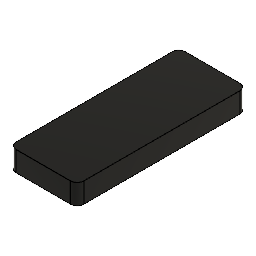
Central Tool Box v19 (Autodesk Fusion 360 archive; units mm, degrees)
design "Soft Spacer"
Autodesk Fusion 360 part; units mm, degrees
sketch "Sketch1" plane through (0, 0, 0) normal (0, 0, 1) x (1, 0, 0)
  line L0 (5, -12.5) -> (-5, -12.5)
  line L1 (-5, -12.5) -> (-5, 12.5)
  line L2 (-5, 12.5) -> (5, 12.5)
  line L3 (5, 12.5) -> (5, -12.5)
  line L4 (5, -12.5) -> (-5, 12.5) construction
  line L5 (-5, -12.5) -> (5, 12.5) construction
  dimension "d1" = 10
  dimension "d2" = 25
  constraint horizontal L0
  constraint perpendicular L0 L1
  constraint parallel L0 L2
  constraint parallel L1 L3
  constraint coincident L4 origin
  constraint coincident L5 origin
  measures "d1" distance of L1.end L2.end
  measures "d2" distance of L0.end L1.end
extrude "Extrude1" add sketch "Sketch1" along normal blind 3
fillet "Fillet1" radius 1 4 edges at (5, -12.5, 1.5) (-5, -12.5, 1.5) (-5, 12.5, 1.5) (5, 12.5, 1.5)

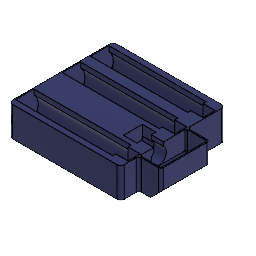
design "CO2 Inflator Holder"
Autodesk Fusion 360 part; units mm, degrees
sketch "Sketch1" plane through (0, 0, 0) normal (0, 0, 1) x (1, 0, 0)
  line L0 (44.5, -42.5) -> (-44.5, -42.5)
  line L1 (-44.5, -42.5) -> (-44.5, 42.5)
  line L2 (-44.5, 42.5) -> (44.5, 42.5)
  line L3 (44.5, 42.5) -> (44.5, -42.5)
  line L4 (44.5, -42.5) -> (-44.5, 42.5) construction
  line L5 (-44.5, -42.5) -> (44.5, 42.5) construction
  dimension "d1" = 85
  dimension "d2" = 89
  constraint horizontal L0
  constraint perpendicular L0 L1
  constraint parallel L0 L2
  constraint parallel L1 L3
  constraint coincident L4 origin
  constraint coincident L5 origin
  measures "d1" distance of L0.end L1.end
  measures "d2" distance of L1.end L2.end
extrude "Extrude1" add sketch "Sketch1" against normal blind 1.2
sketch "Sketch2" plane through (-44.5, 0, 0) normal (-1, 0, 0) x (0, -1, 0)
  line L0 (42.5, 0) -> (-42.5, 0)
  line L1 (-42.5, 0) -> (-42.5, -1.2)
  line L2 (-42.5, -1.2) -> (42.5, -1.2)
  line L3 (42.5, -1.2) -> (42.5, 0)
  line L4 (42.5, 0) -> (42.5, 23.3)
  circle A0 centre (30.5, 11) radius 11
  circle A1 centre (-7.5, 11) radius 11
  circle A2 centre (-30.5, 11) radius 11
  line L5 (38, 23.3) -> (38, 19.0467)
  line L6 (23, 19.0467) -> (23, 23.3)
  line L7 (0, 23.3) -> (0, 19.0467)
  line L8 (-15, 19.0467) -> (-15, 23.3)
  line L9 (-23, 23.3) -> (-23, 19.0467)
  line L10 (-42.5, 0) -> (-42.5, 23.3)
  line L11 (-38, 23.3) -> (-38, 19.0467)
  line L12 (-42.5, 23.3) -> (42.5, 23.3)
  dimension "d5" = 22
  dimension "d7" = 12
  dimension "d10" = 12
  dimension "d12" = 15
  dimension "d17" = 24.5
  dimension "d53" = 38
  constraint coincident L0.start L3.end
  constraint perpendicular L0 L4
  constraint tangent L0 A0
  constraint coincident A0 L5.end
  constraint coincident A0 L6.start
  constraint coincident A1 L7.end
  constraint equal A0 A1
  constraint equal A0 A2
  constraint tangent L0 A1
  constraint tangent L0 A2
  constraint coincident A1 L8.start
  constraint coincident A2 L9.end
  constraint coincident L0.end L1.start
  constraint perpendicular L0 L10
  constraint coincident A2 L11.end
  constraint equal L9 L11
  constraint equal L8 L11
  constraint equal L7 L8
  constraint equal L6 L7
  constraint equal L5 L6
  constraint perpendicular L4 L12
  constraint coincident L5.start L12
  constraint coincident L6.end L12
  constraint coincident L7.start L12
  constraint coincident L8.end L12
  constraint coincident L9.start L12
  constraint coincident L11.start L12
  constraint vertical L5
  constraint vertical L7
  constraint vertical L8
  constraint vertical L9
  constraint vertical L11
  measures "d5" diameter of A0
  measures "d7" distance of L4 A0.centre
  measures "d10" distance of A2.centre L10
  measures "d12" distance of L5 L6
  measures "d17" distance of L2 L12
  measures "d53" distance of A0.centre A1.centre
extrude "Extrude3" add sketch "Sketch2" along normal blind 1
extrude "Extrude4" add sketch "Sketch2" against normal blind 79 contours L0 L4 A0 L5 L12 | L0 A0 A1 L6 L7 L12 | L0 A1 A2 L8 L9 L12 | L0 A2 L10 L11 L12
sketch "Sketch4" plane through (44.5, 0, 0) normal (1, 0, 0) x (0, 1, 0)
  line L0 (42.5, 0) -> (-42.5, 0)
  line L1 (-42.5, 0) -> (-42.5, -1.2)
  line L2 (-42.5, -1.2) -> (42.5, -1.2)
  line L3 (42.5, -1.2) -> (42.5, 0)
  arc A0 (23, 19.0467) -> (30.5, 0) centre (30.5, 11) ccw construction
  arc A1 (30.5, 0) -> (38, 19.0467) centre (30.5, 11) ccw construction
  arc A2 (0, 19.0467) -> (7.5, 0) centre (7.5, 11) ccw construction
  arc A3 (7.5, 0) -> (15, 19.0467) centre (7.5, 11) ccw construction
  arc A4 (-38, 19.0467) -> (-30.5, 0) centre (-30.5, 11) ccw construction
  arc A5 (-30.5, 0) -> (-23, 19.0467) centre (-30.5, 11) ccw construction
  circle A6 centre (30.5, 11) radius 5
  circle A7 centre (7.5, 11) radius 5
  circle A8 centre (-30.5, 11) radius 5
  line L4 (42.5, 0) -> (42.5, 23.3)
  line L5 (-42.5, 23.3) -> (-42.5, 0)
  line L6 (-38, 23.3) -> (-23, 23.3)
  line L7 (-42.5, 23.3) -> (-38, 23.3)
  line L8 (42.5, 23.3) -> (-42.5, 23.3)
  line L9 (-23, 23.3) -> (0, 23.3)
  line L10 (15, 23.3) -> (23, 23.3)
  line L11 (38, 23.3) -> (42.5, 23.3)
  line L12 (35.5, 11) -> (35.5, 27)
  line L13 (25.5, 11) -> (25.5, 27)
  line L14 (12.5, 11) -> (12.5, 23.3)
  line L15 (2.5, 11) -> (2.5, 27)
  line L16 (-25.5, 11) -> (-25.5, 23.3)
  line L17 (-35.5, 11) -> (-35.5, 23.3)
  circle A9 centre (-11.5, 15.05) radius 7.75
  line L18 (-19.25, 15.05) -> (-19.25, 23.3)
  line L19 (-3.75, 15.05) -> (-3.75, 27)
  arc A10 (23, 19.0467) -> (38, 19.0467) centre (30.5, 11) ccw
  arc A11 (0, 19.0467) -> (15, 19.0467) centre (7.5, 11) ccw
  arc A12 (-38, 19.0467) -> (-23, 19.0467) centre (-30.5, 11) ccw
  line L20 (0, 23.3) -> (15, 23.3)
  line L21 (23, 23.3) -> (38, 23.3)
  line L22 (-30.5, 11) -> (7.5, 11) construction
  line L23 (-11.5, 11) -> (-11.5, 15.05) construction
  point P0 (38, 19.0467)
  point P1 (-38, 19.0467)
  point P2 (-23, 19.0467)
  point P3 (38, 19.0467)
  point P4 (-38, 19.0467)
  point P5 (38, 19.0467)
  point P6 (-38, 19.0467)
  dimension "d23" = 10
  dimension "d28" = 15.5
  dimension "d29" = 8.25
  constraint equal A7 A8
  constraint equal A6 A7
  constraint coincident L0.start L3.end
  constraint perpendicular L0 L4
  constraint coincident L0.end L1.start
  constraint coincident L4.end L8.start
  constraint coincident L5.start L7.start
  constraint coincident A6 L12.start
  constraint coincident A6 L13.start
  constraint coincident A7 L14.start
  constraint coincident L6 L14.end
  constraint coincident A7 L15.start
  constraint coincident A8 L16.start
  constraint coincident L6 L16.end
  constraint coincident A8 L17.start
  constraint coincident L6 L17.end
  constraint tangent A6 L13
  constraint tangent A6 L12
  constraint tangent A7 L14
  constraint tangent A7 L15
  constraint tangent A8 L16
  constraint tangent A8 L17
  constraint vertical L17
  constraint vertical L16
  constraint vertical L15
  constraint vertical L14
  constraint vertical L13
  constraint vertical L12
  constraint coincident A9 L18.start
  constraint coincident L6 L18.end
  constraint coincident A9 L19.start
  constraint tangent A9 L19
  constraint tangent A9 L18
  constraint perpendicular L10 L18
  constraint perpendicular L10 L19
  constraint coincident A0.centre A1.centre
  constraint coincident A4.centre A5.centre
  constraint coincident A2.centre A3.centre
  constraint midpoint L22 L23.start
  constraint coincident A9.centre L23.end
  constraint perpendicular L22 L23
  measures "d23" diameter of A6
  measures "d28" diameter of A9
  measures "d29" distance of L6 A9.centre
extrude "Extrude5" add sketch "Sketch4" along normal blind 1
extrude "Extrude6" add sketch "Sketch4" against normal up to surface (10 mm away) contours L0 A6 A7 A8 L4 L5 L6 L7 L8 L9 L10 L11 L12 L13 L14 L15 L16 L17 A9 L18 L19 L20 L21 | L8 L9 A9 L18 L19
extrude "Extrude7" cut sketch "Sketch4" against normal blind 20 contours L8 L9 A9 L18 L19 | A9
sketch "Sketch5" plane through (0, 0, 23.3) normal (0, 0, 1) x (-1, 0, 0)
  line L0 (-44.5, 25.5) -> (-44.5, 35.5)
  line L1 (-45.5, -42.5) -> (45.5, -42.5)
  line L2 (44.5, 38) -> (44.5, 23)
  line L3 (45.5, 42.5) -> (-45.5, 42.5)
  line L4 (-24.5, 19.25) -> (-24.5, 3.75)
  line L5 (-45.5, 42.5) -> (-45.5, -42.5)
  line L6 (-44.5, 35.5) -> (-34.5, 35.5)
  line L7 (-34.5, 35.5) -> (-34.5, 38)
  line L8 (-34.5, 38) -> (44.5, 38)
  line L9 (45.5, -42.5) -> (45.5, 42.5)
  line L10 (44.5, 23) -> (-34.5, 23)
  line L11 (-34.5, 23) -> (-34.5, 25.5)
  line L12 (-34.5, 25.5) -> (-44.5, 25.5)
  line L13 (-34.5, -23) -> (44.5, -23)
  line L14 (44.5, -38) -> (-34.5, -38)
  line L15 (-34.5, -38) -> (-34.5, -35.5)
  line L16 (-34.5, -35.5) -> (-44.5, -35.5)
  line L17 (-44.5, -2.5) -> (-34.5, -2.5)
  line L18 (-34.5, -2.5) -> (-34.5, 0)
  line L19 (-34.5, 0) -> (44.5, 0)
  line L20 (44.5, -15) -> (-34.5, -15)
  line L21 (-35.5, 19.25) -> (-35.5, 3.75)
  line L22 (44.5, 0) -> (44.5, -15)
  line L23 (-44.5, -12.5) -> (-44.5, -2.5)
  line L24 (44.5, -23) -> (44.5, -38)
  line L25 (-44.5, 19.25) -> (-24.5, 19.25)
  line L26 (-24.5, 3.75) -> (-44.5, 3.75)
  line L27 (-44.5, 3.75) -> (-44.5, 19.25)
  line L28 (-34.5, -15) -> (-34.5, -12.5)
  line L29 (-34.5, -12.5) -> (-44.5, -12.5)
  line L30 (-44.5, -25.5) -> (-34.5, -25.5)
  line L31 (-34.5, -25.5) -> (-34.5, -23)
  line L32 (-44.5, -35.5) -> (-44.5, -25.5)
  dimension "d52" = 10
  constraint coincident L21.start L25
  constraint coincident L21.end L26
  measures "d52" distance of L5 L21
extrude "Extrude8" add sketch "Sketch5" against normal up to surface (24.5 mm away) contours L21 L25 L26 L27
sketch "Sketch6" plane through (44.5, 0, 0) normal (-1, 0, 0) x (0, 1, 0)
  line L0 (2.5, -23.3) -> (12.5, -23.3)
  arc A0 (-3.75, -15.05) -> (-19.25, -15.05) centre (-11.5, -15.05) ccw construction
  arc A1 (-3.75, -15.05) -> (-19.25, -15.05) centre (-11.5, -15.05) ccw construction
  circle A2 centre (-11.5, -15.05) radius 6.25
  line L1 (-7.5, -10.2477) -> (-7.5, -23.3)
  line L2 (-15.5, -10.2477) -> (-15.5, -23.3)
  line L3 (2.5, -11) -> (2.5, -23.3)
  line L4 (12.5, -23.3) -> (12.5, -11)
  arc A3 (12.5, -11) -> (2.5, -11) centre (7.5, -11) ccw
  line L5 (25.5, -11) -> (25.5, -23.3)
  line L6 (25.5, -23.3) -> (35.5, -23.3)
  line L7 (35.5, -23.3) -> (35.5, -11)
  arc A4 (35.5, -11) -> (25.5, -11) centre (30.5, -11) ccw
  line L8 (-25.5, -23.3) -> (-25.5, -11)
  arc A5 (-25.5, -11) -> (-35.5, -11) centre (-30.5, -11) ccw
  line L9 (-35.5, -11) -> (-35.5, -23.3)
  line L10 (-35.5, -23.3) -> (-25.5, -23.3)
  line L11 (-15.5, -23.3) -> (-7.5, -23.3)
  point P0 (-3.75, -15.05)
  point P1 (-19.25, -15.05)
  dimension "d35" = 12.5
  dimension "d36" = 8
  constraint concentric A0 A2
  constraint coincident A2 L1.start
  constraint coincident L0 L1.end
  constraint perpendicular L0 L1
  constraint coincident A2 L2.start
  constraint coincident L0 L2.end
  constraint perpendicular L0 L2
  constraint equal L1 L2
  measures "d35" diameter of A2
  measures "d36" distance of L1 L2
extrude "Extrude9" cut sketch "Sketch6" along normal up to surface (9 mm away) and the other way up to surface (1 mm away) contours A2 L1 | A2 L1 L2 | A2 L1 L2 L11 | A2 L2
sketch "Sketch7" plane through (0, 0, 23.3) normal (0, 0, 1) x (-1, 0, 0)
  line L0 (-45.5, -42.5) -> (45.5, -42.5)
  line L1 (44.5, 38) -> (44.5, 23)
  line L2 (45.5, 42.5) -> (-45.5, 42.5)
  line L3 (-44.5, 25.5) -> (-44.5, 35.5)
  line L4 (-45.5, 7.5) -> (-45.5, -42.5)
  line L5 (-44.5, 35.5) -> (-34.5, 35.5)
  line L6 (-34.5, 35.5) -> (-34.5, 38)
  line L7 (-34.5, 38) -> (44.5, 38)
  line L8 (45.5, -42.5) -> (45.5, 42.5)
  line L9 (44.5, 23) -> (-34.5, 23)
  line L10 (-34.5, 23) -> (-34.5, 25.5)
  line L11 (-34.5, 25.5) -> (-44.5, 25.5)
  line L12 (-34.5, -23) -> (44.5, -23)
  line L13 (44.5, -38) -> (-34.5, -38)
  line L14 (-34.5, -38) -> (-34.5, -35.5)
  line L15 (-34.5, -35.5) -> (-44.5, -35.5)
  line L16 (-44.5, -25.5) -> (-34.5, -25.5)
  line L17 (-34.5, -25.5) -> (-34.5, -23)
  line L18 (-44.5, -2.5) -> (-34.5, -2.5)
  line L19 (-34.5, -2.5) -> (-34.5, 0)
  line L20 (-34.5, 0) -> (44.5, 0)
  line L21 (44.5, -15) -> (-34.5, -15)
  line L22 (-34.5, -15) -> (-34.5, -12.5)
  line L23 (-34.5, -12.5) -> (-44.5, -12.5)
  line L24 (-35.5, 19.25) -> (-24.5, 19.25)
  line L25 (-24.5, 19.25) -> (-24.5, 3.75)
  line L26 (-24.5, 3.75) -> (-35.5, 3.75)
  line L27 (-35.5, 15.5) -> (-35.5, 19.25)
  line L28 (44.5, 0) -> (44.5, -15)
  line L29 (-44.5, -12.5) -> (-44.5, -2.5)
  line L30 (44.5, -23) -> (44.5, -38)
  line L31 (-44.5, -35.5) -> (-44.5, -25.5)
  line L32 (-45.5, 26.75) -> (-62.5, 26.75)
  line L33 (-62.5, 26.75) -> (-62.5, -10.75)
  line L34 (-62.5, -10.75) -> (-45.5, -10.75)
  line L35 (-35.5, 7.5) -> (-45.5, 7.5)
  line L36 (-45.5, 42.5) -> (-45.5, 15.5)
  line L37 (-45.5, 15.5) -> (-35.5, 15.5)
  line L38 (-35.5, 3.75) -> (-35.5, 7.5)
  line L39 (-35.5, 17.75) -> (-35.5, 5.25) construction
  line L40 (-35.5, 15.5) -> (-45.5, 15.5) construction
  line L41 (-45.5, 5.25) -> (-45.5, 17.75) construction
  line L42 (-45.5, 7.5) -> (-35.5, 7.5) construction
  line L43 (-45.5, 27.75) -> (-63.5, 27.75)
  line L44 (-63.5, 27.75) -> (-63.5, -11.75)
  line L45 (-63.5, -11.75) -> (-45.5, -11.75)
  dimension "d56" = 17
  dimension "d57" = 9
  dimension "d58" = 16
  dimension "d59" = 1
  dimension "d60" = 1
  dimension "d61" = 1
  constraint coincident L4 L32.start
  constraint perpendicular L4 L32
  constraint perpendicular L32 L33
  constraint coincident L4 L34.end
  constraint perpendicular L4 L34
  constraint coincident L36 L43.start
  constraint perpendicular L36 L43
  constraint perpendicular L43 L44
  constraint coincident L4 L45.end
  constraint perpendicular L4 L45
  measures "d56" distance of L32.start L32.end
  measures "d57" distance of L32 L41.end
  measures "d58" distance of L34 L41.start
  measures "d59" distance of L32 L43
  measures "d60" distance of L33 L44
  measures "d61" distance of L34 L45
extrude "Extrude10" add sketch "Sketch7" against normal up to surface (24.5 mm away) contours L4 L32 L33 L34 L36 L43 L44 L45
sketch "Sketch8" plane through (45.5, 0, 0) normal (1, 0, 0) x (0, 1, 0)
  line L0 (-26.75, 23.3) -> (-26.75, -1.2)
  line L1 (-26.75, -1.2) -> (10.75, -1.2)
  line L2 (10.75, -1.2) -> (10.75, 23.3)
  line L3 (10.75, 23.3) -> (-7.5, 23.3)
  line L4 (-7.5, 23.3) -> (-7.5, 19.8523)
  arc A0 (-15.5, 19.8523) -> (-7.5, 19.8523) centre (-11.5, 15.05) ccw
  line L5 (-15.5, 19.8523) -> (-15.5, 23.3)
  line L6 (-15.5, 23.3) -> (-26.75, 23.3)
  arc A1 (-19.25, 15.05) -> (-3.75, 15.05) centre (-11.5, 15.05) ccw
  arc A2 (-19.25, 15.05) -> (-3.75, 15.05) centre (-11.5, 15.05) ccw
  line L7 (-26.75, 7.3) -> (10.75, 7.3)
  constraint coincident L0 L7.start
  constraint coincident L2 L7.end
  constraint perpendicular L2 L7
  constraint tangent A1 L7
extrude "Extrude11" add sketch "Sketch8" along normal up to surface (17 mm away) contours L0 L1 L2 L7
chamfer "Chamfer1" distance 8.5 angle 45 1 edges at (63.5, -8, -1.2)
fillet "Fillet1" radius 1 4 edges at (45.5, -26.75, 11.05) (62.5, -26.75, 11.05) (62.5, 10.75, 11.05) (45.5, 10.75, 11.05)
fillet "Fillet4" radius 2 4 edges at (45.5, -27.75, 11.05) (63.5, -27.75, 11.05) (63.5, 11.75, 11.05) (45.5, 11.75, 11.05)
fillet "Fillet5" radius 1 8 edges at (45.7929, 10.4571, 7.3) (54, 10.75, 7.3) (62.2071, 10.4571, 7.3) (62.5, -8, 7.3) (62.2071, -26.4571, 7.3) (54, -26.75, 7.3) (45.7929, -26.4571, 7.3) (45.5, -8, 7.3)
fillet "Fillet2" radius 3 4 edges at (45.5, 42.5, 11.05) (45.5, -42.5, 11.05) (-45.5, 42.5, 11.05) (-45.5, -42.5, 11.05)

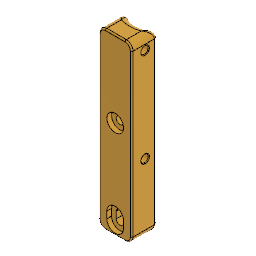
design "Connector"
Autodesk Fusion 360 part; units mm, degrees
sketch "Sketch1" plane through (0, 0, 0) normal (0, 1, 0) x (1, 0, 0)
  line L0 (12.3, 65) -> (-12.3, 65)
  line L1 (-12.3, 65) -> (-12.3, -65)
  line L2 (-12.3, -65) -> (12.3, -65)
  line L3 (12.3, -65) -> (12.3, 65)
  line L4 (12.3, 65) -> (-12.3, -65) construction
  line L5 (-12.3, 65) -> (12.3, -65) construction
  dimension "d1" = 24.6
  dimension "d2" = 130
  constraint horizontal L0
  constraint perpendicular L0 L1
  constraint parallel L0 L2
  constraint parallel L1 L3
  constraint coincident L4 origin
  constraint coincident L5 origin
  measures "d1" distance of L1.end L2.end
  measures "d2" distance of L0.end L1.end
extrude "Extrude1" add sketch "Sketch1" along normal blind 20
sketch "Sketch2" plane through (0, 20, 0) normal (0, 1, 0) x (-1, 0, 0)
  line L0 (-12.3, 65) -> (-12.3, -65)
  line L1 (-12.3, -65) -> (12.3, -65)
  line L2 (12.3, -65) -> (12.3, 65)
  line L3 (12.3, 65) -> (-12.3, 65)
  arc A0 (-2.75, -57) -> (2.75, -57) centre (0, -57) ccw
  arc A1 (2.75, -52) -> (-2.75, -52) centre (0, -52) ccw
  line L4 (2.75, -52) -> (2.75, -57)
  line L5 (-2.75, -52) -> (-2.75, -57)
  line L6 (0, 0) -> (0, 8) construction
  circle A2 centre (0, 8) radius 2.75
  dimension "d5" = 5.5
  dimension "d6" = 5
  dimension "d7" = 60
  dimension "d8" = 8
  constraint tangent A0 L4
  constraint tangent A0 L5
  constraint tangent A1 L5
  constraint tangent A1 L4
  constraint coincident L6.start origin
  constraint parallel L2 L6
  constraint coincident L6.end A2.centre
  constraint equal A1 A2
  constraint coincident A1.centre L6
  constraint coincident A0.centre L6
  constraint equal A0 A1
  measures "d5" diameter of A2
  measures "d6" distance of A0.centre A1.centre
  measures "d7" distance of A1.centre L6.end
  measures "d8" distance of L1 A0.centre
extrude "Extrude2" cut sketch "Sketch2" against normal up to surface (20 mm away) contours A0 A1 L4 L5 | A2
sketch "Sketch3" plane through (0, 0, 0) normal (0, -1, 0) x (1, 0, 0)
  line L0 (-2.75, -57) -> (-2.75, -52)
  arc A0 (2.75, -52) -> (-2.75, -52) centre (0, -52) ccw
  line L1 (2.75, -52) -> (2.75, -57)
  arc A1 (-2.75, -57) -> (2.75, -57) centre (0, -57) ccw
  circle A2 centre (0, 8) radius 2.75
  line L2 (12.3, -65) -> (12.3, 65)
  line L3 (12.3, 65) -> (-12.3, 65)
  line L4 (-12.3, 65) -> (-12.3, -65)
  line L5 (-12.3, -65) -> (12.3, -65)
  line L6 (-6.25, -57) -> (-6.25, -52)
  arc A3 (6.25, -52) -> (-6.25, -52) centre (0, -52) ccw
  line L7 (6.25, -52) -> (6.25, -57)
  arc A4 (-6.25, -57) -> (6.25, -57) centre (0, -57) ccw
  circle A5 centre (0, 8) radius 6.25
  dimension "d11" = 3.5
  constraint concentric A2 A5
  constraint equal A3 A5
extrude "Extrude3" cut sketch "Sketch3" against normal blind 3.5 contours L6 A3 L7 A4 | A5
sketch "Sketch4" plane through (12.3, 0, 0) normal (1, 0, 0) x (0, 1, 0)
  line L0 (0, 65) -> (0, -65)
  line L1 (0, -65) -> (20, -65)
  line L2 (20, -65) -> (20, 65)
  line L3 (20, 65) -> (0, 65)
  line L4 (10, 65) -> (10, -48.6514) construction
  circle A0 centre (10, 56) radius 2.75
  circle A1 centre (10, -14) radius 2.75
  dimension "d14" = 5.5
  dimension "d15" = 70
  dimension "d16" = 51
  constraint midpoint L3 L4.start
  constraint perpendicular L3 L4
  constraint coincident L4 A0.centre
  constraint coincident L4 A1.centre
  constraint equal A0 A1
  measures "d14" diameter of A0
  measures "d15" distance of A0.centre A1.centre
  measures "d16" distance of L1 A1.centre
extrude "Extrude4" cut sketch "Sketch4" against normal up to surface (24.6 mm away) contours A0 | A1
chamfer "Chamfer1" distance 0.5 angle 45 4 edges at (-12.3, 7.4361, -14.9944) (-12.3, 7.4361, 55.0056) (12.3, 7.4361, -13.0056) (12.3, 7.4361, 56.9944)
sketch "Sketch5" plane through (0, 0, -65) normal (0, 0, -1) x (1, 0, 0)
  line L0 (12.3, 0) -> (-12.3, 0)
  line L1 (-12.3, 0) -> (-12.3, -20)
  line L2 (-12.3, -20) -> (12.3, -20)
  line L3 (12.3, -20) -> (12.3, 0)
  line L4 (-12.3, -20) -> (-12.3, -21.3813)
  line L5 (12.3, -20) -> (12.3, -21.3798)
  line L6 (12.3, -15.75) -> (-12.3, -15.75) construction
  arc A0 (12.3, -21.3798) -> (-12.3, -21.3813) centre (0.0007, -32) ccw
  line L7 (-11.8, -12.75) -> (-11.8, -7.25)
  line L8 (11.8, -7.25) -> (11.8, -12.75)
  line L9 (11.8, -12.75) -> (-11.8, -12.75) construction
  dimension "d37" = 3
  dimension "d40" = 16.25
  constraint coincident L1.end L2.start
  constraint perpendicular L2 L4
  constraint coincident L2.end L3.start
  constraint perpendicular L2 L5
  constraint coincident L5 L6.start
  constraint coincident L4 L6.end
  constraint perpendicular L4 L6
  constraint tangent L6 A0
  constraint coincident L8.end L9.start
  constraint coincident L7.start L9.end
  measures "d37" distance of L6 L9
  measures "d40" radius of A0
extrude "Extrude5" add sketch "Sketch5" against normal up to surface (130 mm away) contours L2 L5 A0 | L2 L4 A0
extrude "Extrude8" cut sketch "Sketch5" against normal up to surface (130 mm away) contours L2 A0
fillet "Fillet4" radius 2 2 edges at (-12.3, 21.3813, 0) (12.3, 21.3798, 0)
fillet "Fillet1" radius 5 4 edges at (12.3, 10, -65) (-12.3, 10, -65) (12.3, 10, 65) (-12.3, 10, 65)
fillet "Fillet3" radius 1 8 edges at (0, 0, -65) (-10.8355, 0, -63.5355) (-12.3, 0, 0) (-10.8355, 0, 63.5355) (0, 0, 65) (10.8355, 0, 63.5355) (12.3, 0, 0) (10.8355, 0, -63.5355)
extrude "Extrude7" cut sketch "Sketch3" along normal up to surface (35.75 mm away) from surface at -50 contours L0 A0 L1 A1 | A2 | L6 A3 L7 A4 | A5
equation "d40 = ( 32.5 / 2 ) * 1 mm"

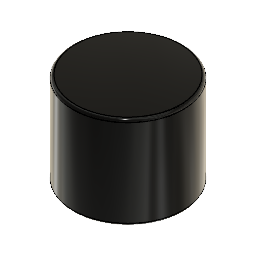
design "Nut Cover"
Autodesk Fusion 360 part; units mm, degrees
sketch "Sketch1" plane through (0, 0, 0) normal (0, 0, 1) x (1, 0, 0)
  circle A0 centre (0, 0) radius 5.95
  circle A1 centre (0, 0) radius 3
  dimension "d1" = 11.9
  dimension "d2" = 6
  constraint coincident A0.centre A1.centre
  constraint concentric A0 A1
  measures "d1" diameter of A0
  measures "d2" diameter of A1
extrude "Extrude1" add sketch "Sketch1" against normal blind 5
extrude "Extrude2" add sketch "Sketch1" along normal blind 5 contours A0 | A1
fillet "Fillet1" radius 0.3 2 edges at (-5.5473, 2.1516, -5) (-5.5473, -2.1516, 5)
